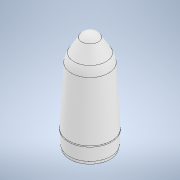
# Autodesk Inventor part: Upper-Threaded-v2
Saved by Autodesk Inventor 2022 (Build 260153000, 153)
## iProperties
Created: 2021-08-11
Part Number: Upper-Threaded-v2
Material: Polycarbonate, Smoke
Document SubType Name: Modeling
Designer: incep
Density: 1.2 g/cm^3
Appearance: Polycarbonate - Smoked
Author: incep
Autodesk Inventor part; units mm, degrees
ref_plane "YZ Plane" through (0, 0, 0) normal (1, 0, 0) x (0, 1, 0)
ref_plane "XZ Plane" through (0, 0, 0) normal (0, 1, 0) x (-1, 0, 0)
ref_plane "XY Plane" through (0, 0, 0) normal (0, 0, 1) x (1, 0, 0)
sketch "Bulb Copy" plane through (0, 0, 0) normal (0, 0, 1) x (1, 0, 0)
  line L0 (-16.5, 55) -> (16.5, 55) construction
  line L1 (16.5, 55) -> (16.5, 0)
  line L2 (16.5, 0) -> (-16.5, 0)
  line L3 (-16.5, 0) -> (-16.5, 55)
  line L4 (-10.5, 63) -> (10.5, 63)
  line L5 (10.5, 63) -> (10.5, 55) construction
  line L6 (10.5, 55) -> (-10.5, 55) construction
  line L7 (-10.5, 55) -> (-10.5, 63) construction
  line L8 (-16.5, 55) -> (-10.5, 63)
  line L9 (10.5, 63) -> (16.5, 55)
  line L10 (0, 63) -> (0, 0)
  point P0 (0, 55)
  dimension "d0" = 33
  dimension "d1" = 55
  dimension "d2" = 21
  dimension "d3" = 63
  constraints: 22 end point, 4 parallel, 2 horizontal, 2 midpoint, 2 perpendicular, 1 collinear, 1 vertical, 1 vertical alignment
  measures "d0" distance of L1.end L2.end
  measures "d1" distance of L0.end L1.end
  measures "d2" distance of L4.start L4.end
  measures "d3" distance from line of L10.end L4
sketch "Top Sketch" plane through (0, 0, 0) normal (0, 0, 1) x (1, 0, 0)
  line L0 (-17.5, 56) -> (17.5, 56) construction
  line L1 (17.5, 56) -> (17.5, -17) construction
  line L2 (17.5, -17) -> (-17.5, -17) construction
  line L3 (-17.5, -17) -> (-17.5, 56) construction
  line L4 (16.5, 55) -> (16.5, 0) projected
  line L5 (-16.5, 0) -> (-16.5, 55) projected
  line L6 (-19.5, 58) -> (19.5, 58) construction
  line L7 (19.5, 58) -> (19.5, -17) construction
  line L8 (19.5, -17) -> (-19.5, -17) construction
  line L9 (-19.5, -17) -> (-19.5, 58) construction
  line L10 (-22.5, 61) -> (22.5, 61) construction
  line L11 (22.5, 61) -> (22.5, -17) construction
  line L12 (22.5, -17) -> (-22.5, -17) construction
  line L13 (-22.5, -17) -> (-22.5, 61) construction
  line L14 (-10.5, 63) -> (10.5, 63) projected
  line L15 (-16.5, 55) -> (16.5, 55) construction
  line L16 (-22.5, 0) -> (-19.1379, 65) construction
  line L17 (22.5, 0) -> (19.1379, 65) construction
  line L18 (-19.1379, 65) -> (19.1379, 65) construction
  line L19 (-19.1379, 65) -> (0, 97.878) construction
  line L20 (0, 97.878) -> (19.1379, 65) construction
  line L21 (-16.5, 55) -> (-10.5, 63) projected
  line L22 (-22.4714, 0.552) -> (-19.3883, 60.1601)
  line L23 (-16.6999, 69.1884) -> (-8.6425, 83.0307)
  line L24 (8.6425, 83.0307) -> (16.6999, 69.1884)
  line L25 (19.3883, 60.1601) -> (22.4714, 0.552)
  arc A0 (-16.6999, 69.1884) -> (-19.3883, 60.1601) centre (0.585, 59.127) ccw
  arc A1 (19.3883, 60.1601) -> (16.6999, 69.1884) centre (-0.585, 59.127) ccw
  arc A2 (8.6425, 83.0307) -> (-8.6425, 83.0307) centre (0, 78) ccw
  line L26 (-22.4675, -0.5518) -> (-21.6768, -13.9952)
  line L27 (22.4675, -0.5518) -> (21.5, -17)
  arc A3 (-22.4714, 0.552) -> (-22.4675, -0.5518) centre (-12.4848, 0.0354) ccw
  arc A4 (22.4675, -0.5518) -> (22.4714, 0.552) centre (12.4848, 0.0354) ccw
  line L28 (-17.5, 56) -> (-11.0463, 64.605)
  line L29 (-10.75, 65) -> (10.75, 65) construction
  line L30 (11.0463, 64.605) -> (17.5, 56)
  line L31 (10.5, 63) -> (16.5, 55) projected
  line L32 (0, -17) -> (0, 88) construction
  line L33 (17.5, -10) -> (-17.5, -10)
  line L34 (-17.5, 56) -> (-17.5, -10)
  line L35 (17.5, 56) -> (17.5, -10)
  line L36 (0, 88) -> (0, -17)
  line L37 (10.75, 65) -> (0, 76.7219) construction
  line L38 (0, 76.7219) -> (-10.75, 65) construction
  line L39 (10.4163, 65.3639) -> (7.37, 68.6856)
  line L40 (-7.37, 68.6856) -> (-10.4163, 65.3639)
  arc A5 (11.0463, 64.605) -> (10.4163, 65.3639) centre (3.0463, 58.605) ccw
  arc A6 (-10.4163, 65.3639) -> (-11.0463, 64.605) centre (-3.0463, 58.605) ccw
  arc A7 (7.37, 68.6856) -> (-7.37, 68.6856) centre (0, 61.9267) ccw
  line L41 (-17, 0) -> (-17, -31.7952) construction
  line L42 (-17, -31.7952) -> (17, -31.7952) construction
  line L43 (17, -31.7952) -> (17, 0) construction
  line L44 (14.5, 12.1752) -> (-14.5, 12.1752) construction
  line L45 (6.5, 0) -> (-6.5, 0) construction
  line L46 (-6.5, 0) -> (-6.5, -37) construction
  line L47 (-6.5, -37) -> (6.5, -37) construction
  line L48 (6.5, -37) -> (6.5, 0) construction
  line L49 (-6.5, -37) -> (-16.032, -24.2907) construction
  arc A8 (-21.6768, -13.9952) -> (-21.0266, -17) centre (-11.694, -13.408) ccw
  line L50 (0, -17) -> (-21.0266, -17)
  point P0 (0, 0)
  point P1 (-21.5, -17)
  point P2 (0, -10)
  point P3 (0, 65)
  point P4 (0, 71.9267)
  point P5 (0, 0)
  point P6 (0, -12.9338)
  point P7 (0, 0)
  point P8 (0, 12.1752)
  point P9 (0, -17)
  dimension "d4" = 1
  dimension "d5" = 2
  dimension "d6" = 3
  dimension "d7" = 17
  dimension "d9" = 1
  dimension "d10" = 2
  dimension "d11" = 3
  dimension "d13" = 2
  dimension "d14" = 20
  dimension "d15" = 20
  dimension "d16" = 10
  dimension "d17" = 1
  dimension "d18" = 1
  dimension "d19" = 10
  dimension "d20" = 10
  dimension "d22" = 10
  dimension "d39" = 33
  dimension "d42" = 10
  dimension "d43" = 10
  dimension "d44" = 10
  dimension "d45" = 34
  dimension "d46" = 29
  dimension "d56" = 88
  dimension "d64" = 13
  dimension "d65" = 37
  dimension "d66" = 10
  dimension "d268" = 35
  constraints: 90 end point, 27 point on line, 19 point on circle, 18 tangent, 11 parallel, 9 centre point, 7 collinear, 7 vertical alignment, 6 horizontal, 5 midpoint, 4 coincident, 4 perpendicular, 2 horizontal alignment
  measures "d4" distance between parallel lines of L1 L4
  measures "d5" distance between parallel lines of L7 L1
  measures "d6" distance between parallel lines of L11 L7
  measures "d7" distance of point (0, -17) point (0, 0)
  measures "d9" distance between parallel lines of L15 L0
  measures "d10" distance between parallel lines of L0 L6
  measures "d11" distance between parallel lines of L6 L10
  measures "d13" distance between parallel lines of L14 L18
  measures "d14" radius of A0
  measures "d15" radius of A1
  measures "d16" radius of A2
  measures "d17" distance of point (-21.5, -17) L12.end
  measures "d18" distance of L11.end L27.end
  measures "d19" radius of A3
  measures "d20" radius of A4
  measures "d22" vertical distance of point (0, 0) L33.start
  measures "d39" distance between parallel lines of L5 L4
  measures "d42" radius of A5
  measures "d43" radius of A6
  measures "d44" radius of A7
  measures "d45" distance of L43.end L41.start
  measures "d46" distance of L44.start L44.end
  measures "d56" distance of L32.end point (0, 0)
  measures "d64" distance of L46.end L47.end
  measures "d65" distance of L45.end L46.end
  measures "d66" radius of A8
  measures "d268" distance of L33.start L33.end
revolve "Top" add sketch "Top Sketch" angle 360 about axis through (0, 88, 0) along (0, -1, 0) contours L22 A0 L23 A2 L36 A7 L40 A6 L28 L34 L33 L50 A8 L26 A3
sketch "Sketch6" plane through (0, -17, 0) normal (0, -1, 0) x (1, 0, 0)
  circle A0 centre (0, 0) radius 3.2051 construction
  point P0 (0, 0)
  constraints: 1 centre point, 1 coincident
hole "Hole3" at (0, -17, 0) direction (0, 1, 0) diameter 39.84 depth 8 tip angle 90
thread "Thread9" size "M42x2" class "6H" standard "ANSI Metric M Profile" length 8
sketch "Sketch22" plane through (0, -17, 0) normal (-1, 0, 0) x (0, 0, 1)
  line L0 (19.92, 0) -> (19.92, 8)
  line L1 (19.92, 8) -> (18.8375, 8)
  line L2 (18.8375, 8) -> (18.8375, 0)
  line L3 (18.8375, 0) -> (19.92, 0)
  line L4 (0, -16) -> (0, 96) projected
  constraints: 8 end point
revolve "Revolution12" add sketch "Sketch22" angle 360 about axis through (0, -17, 0) along (0, 1, 0) separate body
sketch "Sketch21" plane through (0, -17, 19.92) normal (1, 0, 0) x (0, 1, 0)
  line L0 (-1, 0.433) -> (-1.3222, -0.125) construction
  line L1 (-1, 0.433) -> (-0.6778, -0.125) construction
  line L2 (-1, 0.433) -> (-1, 0) construction
  line L3 (-1.25, 0) -> (-1.1057, 0) construction
  line L4 (0, -1.299) -> (0.125, -1.0825) construction
  line L5 (-2, -1.299) -> (-2.125, -1.0825) construction
  line L6 (-2.125, -1.0825) -> (-2, -1.0825) construction
  line L7 (-1.875, -1.0825) -> (-2, -1.299) construction
  arc A0 (-1.1057, 0) -> (-1.3222, -0.125) centre (-1.1057, -0.25) ccw
  arc A1 (-0.6778, -0.125) -> (-0.8943, 0) centre (-0.8943, -0.25) ccw
  line L8 (0, -1.299) -> (0, -1.0825) construction
  line L9 (-2, -1.299) -> (-2, -1.0825) construction
  arc A2 (-0.1611, -1.02) -> (-0.0528, -1.0825) centre (-0.0528, -0.9575) ccw
  line L10 (-0.6778, -0.125) -> (-0.1611, -1.02)
  line L11 (-1.1057, 0) -> (-0.8943, 0)
  line L12 (-1.3222, -0.125) -> (-1.8389, -1.02)
  line L13 (-0.0528, -1.0825) -> (0, -1.0825) construction
  line L14 (0, -1.0825) -> (0.125, -1.0825) construction
  arc A3 (-1.9472, -1.0825) -> (-1.8389, -1.02) centre (-1.9472, -0.9575) ccw
  line L15 (-1.8389, -1.02) -> (-1.875, -1.0825) construction
  line L16 (-2, -1.0825) -> (-1.9472, -1.0825) construction
  line L17 (-1.9472, -1.0825) -> (-0.0528, -1.0825)
  line L18 (0, 0) -> (0.4413, 0)
  line L19 (0, 0) -> (0, 0.419)
  line L20 (0, -1.299) -> (-0.1611, -1.02) construction
  dimension "d247" = 0.433
  dimension "d248" = 0.25
  dimension "d249" = 0.125
  dimension "d250" = 0.2165
  dimension "d251" = 2
  dimension "Sketch21_MajorRadius" = 1.0825
  dimension "d253" = 60
  dimension "Sketch21_ThreadOffset" = 0
  dimension "Sketch21_MinorRadius" = 0
  constraints: 42 end point, 17 tangent, 8 point on circle, 6 parallel, 5 collinear, 4 centre point, 3 point on line, 3 vertical, 2 equal radius, 2 horizontal, 2 perpendicular, 1 equal length, 1 midpoint, 4 other
  measures "d247" distance from line of L0.start L3
  measures "d248" radius of A0
  measures "d249" radius of A2
  measures "d250" distance from line of L14 L4.start
  measures "d251" distance between parallel lines of L8 L9
  measures "Sketch21_MajorRadius" distance between parallel lines of L14 L18
  measures "d253" angle of L10 L12
  measures "Sketch21_ThreadOffset" distance between parallel lines of L19 L8
  measures "Sketch21_MinorRadius" distance between parallel lines of L18 L11
coil "Coil8" sketch "Sketch21" operation cut axis through (0, -17, 0) along (0, 1, 0) pitch 2.002 turns 5.994006 hand right bodies 2
equation "\"d92\" = 0.1875"
equation "\"Sketch7_Pitch\" = 1.5"
equation "\"d94\" = 60deg"
equation "\"d120\" = 0.25"
equation "\"Sketch9_Pitch\" = 2"
equation "\"d122\" = 60deg"
equation "\"d141\" = 0.1875"
equation "\"Sketch11_Pitch\" = 1.5"
equation "\"d143\" = 60deg"
equation "\"d164\" = 0.25"
equation "\"Sketch13_Pitch\" = 2"
equation "\"d166\" = 60deg"
equation "\"d187\" = 0.375"
equation "\"Sketch15_Pitch\" = 3"
equation "\"d189\" = 60deg"
equation "\"d210\" = 0.25"
equation "\"Sketch17_Pitch\" = 2"
equation "\"d212\" = 60deg"
equation "\"d233\" = 0.25"
equation "\"Sketch19_Pitch\" = 2"
equation "\"d235\" = 60deg"
equation "\"d256\" = 0.25"
equation "\"Sketch21_Pitch\" = 2"
equation "\"d258\" = 60deg"
body "Solid2"
body "Solid10"
